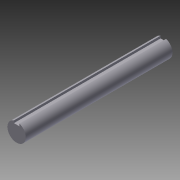
# Autodesk Inventor part: Ad-Hoc 5!8 keyed axle
Saved by Autodesk Inventor 2011 SP1 (Build 150282100, 282)
## iProperties
Created: 2011-01-12
Part Number: Ad-Hoc 5!8 keyed axle
Document SubType Name: Modeling
Designer: Christopher
Density: 1 g/cm^3
Author: Christopher
Autodesk Inventor part; units mm, degrees
ref_plane "YZ Plane" through (0, 0, 0) normal (1, 0, 0) x (0, 1, 0)
ref_plane "XZ Plane" through (0, 0, 0) normal (0, 1, 0) x (-1, 0, 0)
ref_plane "XY Plane" through (0, 0, 0) normal (0, 0, 1) x (1, 0, 0)
sketch "Sketch1" plane through (0, 0, 0) normal (0, 0, 1) x (1, 0, 0)
  circle A0 centre (0, 0) radius 7.9375
  line L0 (0, 7.9375) -> (0, 5.5562)
  line L1 (0, 5.5562) -> (2.3813, 5.5563)
  line L2 (2.3813, 5.5563) -> (2.3813, 7.9375)
  line L3 (2.3813, 7.9375) -> (0, 7.9375)
  line L4 (0, 5.5562) -> (-2.3812, 5.5562)
  line L5 (0, 7.9375) -> (-2.3813, 7.9375)
  line L6 (-2.3813, 7.9375) -> (-2.3812, 5.5562)
  line L7 (-2.3813, 7.5719) -> (-2.3812, 5.5562)
  line L8 (2.3813, 5.5563) -> (2.3813, 7.5719)
  dimension "d0" = 15.875
  dimension "d1" = 2.3813
  dimension "d2" = 2.3813
  dimension "d3" = 2.3813
  constraints: 18 end point, 4 parallel, 4 point on circle, 2 perpendicular, 2 point on line, 1 centre point, 1 coincident, 1 collinear, 1 tangent, 1 vertical
  measures "d0" diameter of A0
  measures "d1" distance of L0.start L0.end
  measures "d2" distance between parallel lines of L0 L6
  measures "d3" distance between parallel lines of L2 L0
extrude "Extrusion1" add sketch "Sketch1" against normal blind 127 contours A0 L6 L4 L1 L2
body "Solid1"
